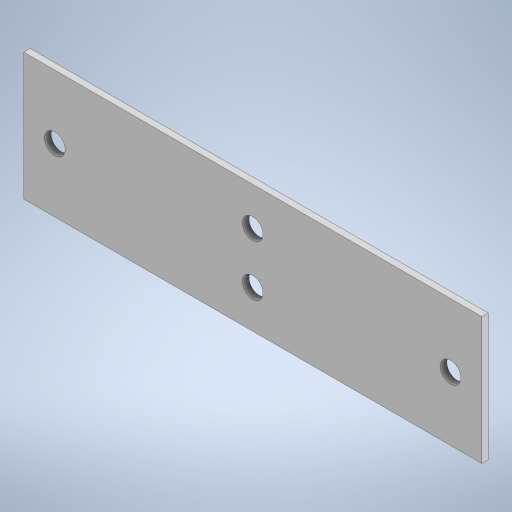
# Autodesk Inventor part: side2
Saved by Autodesk Inventor 2023 (Build 270158000, 158)
## iProperties
Created: 2023-05-28
Part Number: side2
Material: 一般
Document SubType Name: Sheet Metal
Designer: 310611102
Density: 1 g/cm^3
Sheet Metal Rule: Default_mm
Appearance: 預設
Author: 310611102
Autodesk Inventor part; units mm, degrees
ref_plane "YZ Plane" through (0, 0, 0) normal (1, 0, 0) x (0, 1, 0)
ref_plane "XZ Plane" through (0, 0, 0) normal (0, 1, 0) x (-1, 0, 0)
ref_plane "XY Plane" through (0, 0, 0) normal (0, 0, 1) x (1, 0, 0)
sketch "Sketch1" plane through (0, 0, 0) normal (0, 0, 1) x (1, 0, 0)
  line L0 (-36, 10) -> (36, 10)
  line L1 (36, 10) -> (36, -10)
  line L2 (36, -10) -> (-36, -10)
  line L3 (-36, -10) -> (-36, 10)
  line L4 (-36, 10) -> (36, -10) construction
  line L5 (36, 10) -> (-36, -10) construction
  circle A0 centre (31.1, 0) radius 1.6
  line L6 (0, 0) -> (12.8976, 0)
  line L7 (0, 0) -> (0, 11.3109)
  circle A1 centre (-31.1, 0) radius 1.6
  circle A2 centre (0, 4) radius 1.6
  circle A3 centre (0, -4) radius 1.6
  dimension "d0" = 72
  dimension "d1" = 20
  dimension "d2" = 3.2
  dimension "d3" = 4.9
  dimension "d11" = 3.2
  dimension "d12" = 6
  measures "d0" distance of L1.end L2.end
  measures "d1" distance of L0.end L1.end
  measures "d2" diameter of A0
  measures "d3" distance from line of L1 A0.centre
  measures "d11" diameter of A2
  measures "d12" distance from line of L0 A2.centre
sketch "Sketch2" plane through (0, 0, 1) normal (0, 0, 1) x (1, 0, 0)
  line L0 (-17.5, 32.5) -> (-12.5, 32.5)
  line L1 (-7.5, 27.5) -> (-7.5, 12.5)
  line L2 (-12.5, 7.5) -> (-17.5, 7.5)
  line L3 (-22.5, 12.5) -> (-22.5, 27.5)
  line L4 (-22.5, 32.5) -> (-7.5, 7.5) construction
  line L5 (-7.5, 32.5) -> (-22.5, 7.5) construction
  line L6 (0, 16.0345) -> (0, -16.0345)
  line L7 (-10.8621, 0) -> (10.8621, 0)
  arc A0 (-17.5, 32.5) -> (-22.5, 27.5) centre (-17.5, 27.5) ccw
  arc A1 (-7.5, 27.5) -> (-12.5, 32.5) centre (-12.5, 27.5) ccw
  arc A2 (-12.5, 7.5) -> (-7.5, 12.5) centre (-12.5, 12.5) ccw
  arc A3 (-22.5, 12.5) -> (-17.5, 7.5) centre (-17.5, 12.5) ccw
  line L8 (17.5, 32.5) -> (12.5, 32.5)
  line L9 (7.5, 27.5) -> (7.5, 12.5)
  line L10 (12.5, 7.5) -> (17.5, 7.5)
  line L11 (22.5, 12.5) -> (22.5, 27.5)
  line L12 (22.5, 32.5) -> (7.5, 7.5) construction
  line L13 (7.5, 32.5) -> (22.5, 7.5) construction
  arc A4 (22.5, 27.5) -> (17.5, 32.5) centre (17.5, 27.5) ccw
  arc A5 (12.5, 32.5) -> (7.5, 27.5) centre (12.5, 27.5) ccw
  arc A6 (7.5, 12.5) -> (12.5, 7.5) centre (12.5, 12.5) ccw
  arc A7 (17.5, 7.5) -> (22.5, 12.5) centre (17.5, 12.5) ccw
  line L14 (-17.5, -32.5) -> (-12.5, -32.5)
  line L15 (-7.5, -27.5) -> (-7.5, -12.5)
  line L16 (-12.5, -7.5) -> (-17.5, -7.5)
  line L17 (-22.5, -12.5) -> (-22.5, -27.5)
  line L18 (-22.5, -32.5) -> (-7.5, -7.5) construction
  line L19 (-7.5, -32.5) -> (-22.5, -7.5) construction
  arc A8 (-22.5, -27.5) -> (-17.5, -32.5) centre (-17.5, -27.5) ccw
  arc A9 (-12.5, -32.5) -> (-7.5, -27.5) centre (-12.5, -27.5) ccw
  arc A10 (-7.5, -12.5) -> (-12.5, -7.5) centre (-12.5, -12.5) ccw
  arc A11 (-17.5, -7.5) -> (-22.5, -12.5) centre (-17.5, -12.5) ccw
  arc A12 (12.5, -7.5) -> (7.5, -12.5) centre (12.5, -12.5) ccw
  line L20 (12.5, -7.5) -> (17.5, -7.5)
  arc A13 (22.5, -12.5) -> (17.5, -7.5) centre (17.5, -12.5) ccw
  line L21 (7.5, -27.5) -> (7.5, -12.5)
  line L22 (22.5, -12.5) -> (22.5, -27.5)
  arc A14 (7.5, -27.5) -> (12.5, -32.5) centre (12.5, -27.5) ccw
  line L23 (7.5, -32.5) -> (22.5, -7.5) construction
  line L24 (22.5, -32.5) -> (7.5, -7.5) construction
  line L25 (17.5, -32.5) -> (12.5, -32.5)
  arc A15 (17.5, -32.5) -> (22.5, -27.5) centre (17.5, -27.5) ccw
  point P0 (0, 0)
  point P1 (-15, 20)
  point P2 (0, 0)
  point P3 (15, 20)
  point P4 (-15, -20)
  point P5 (15, -20)
  dimension "d13" = 15
  dimension "d14" = 15
  dimension "d15" = 15
  dimension "d16" = 25
  dimension "d17" = 5
  constraints: 52 end point, 51 symmetric about line, 32 point on circle, 32 point on line, 16 centre point, 8 tangent, 4 midpoint, 3 equal radius, 2 horizontal, 2 parallel, 1 coincident, 1 perpendicular, 1 vertical, 12 other
  measures "d13" distance of L4.start L5.start
  measures "d14" diameter of L1 L6
  measures "d15" diameter of L2 L7
  measures "d16" distance of L5.start L4.end
  measures "d17" radius of A0
extrude "Plate1" add sketch "Sketch1" along normal blind 1
equation "\"d5\" = 厚度"
equation "\"折彎半徑\" = 厚度"
equation "\"折彎離隙寬度\" = 厚度"
equation "\"折彎離隙深度\" = 0.5 * 厚度"
equation "\"轉角離隙大小\" = 4 * 厚度"
equation "\"最小剩餘\" = 2 * 厚度"
equation "\"轉移半徑\" = 折彎半徑"
equation "\"Jacobi半徑大小\" = 折彎半徑"
equation "\"間隙大小\" = 厚度"
equation "\"厚度\" = 1"
body "Solid1"
